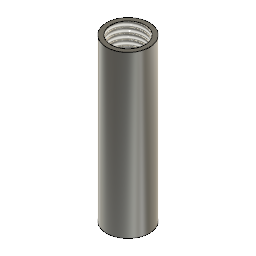
pen_part1 (Autodesk Fusion 360 design; units mm, degrees)
Autodesk Fusion 360 part; units mm, degrees
cylinder "CylinderPrimitive1" add diameter 12 height 45 placed x (1, 0, 0) y (0, 1, 0) z (0, 0, 1) at (0, 0, 0)
sketch "Sketch2" plane through (0, 0, 45) normal (0, 0, 1) x (-1, 0, 0)
  circle A0 centre (0, 0) radius 6
  circle A1 centre (0, 0) radius 4.75
  dimension "d3" = 9.5
  constraint coincident A0.centre A1.centre
  measures "d3" diameter of A1
extrude "Extrude1" cut sketch "Sketch2" against normal blind 40 contours A1
thread "Thread1" "ISO Metric profile 11.0 M11x1.5 6H" major diameter 11.1933 minor diameter 9.5262 pitch 1.5 angle 60 resizes the face on face at (-4.7441, 0.2368, 18.3333)
